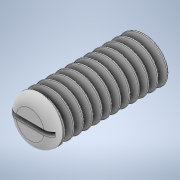
# Autodesk Inventor part: Tornillo de presion punta fuerte
Saved by Autodesk Inventor 2020 (Build 240168000, 168)
## iProperties
Created: 2020-09-17
Part Number: Tornillo de presion punta fuerte
Material: Generic
Document SubType Name: Modeling
Designer: aaron
Density: 1 g/cm^3
Appearance: Default
Author: aaron
Autodesk Inventor part; units mm, degrees
ref_plane "YZ Plane" through (0, 0, 0) normal (1, 0, 0) x (0, 1, 0)
ref_plane "XZ Plane" through (0, 0, 0) normal (0, 1, 0) x (-1, 0, 0)
ref_plane "XY Plane" through (0, 0, 0) normal (0, 0, 1) x (1, 0, 0)
sketch "Sketch1" plane through (0, 0, 0) normal (0, 0, 1) x (1, 0, 0)
  circle A0 centre (0, 0) radius 3.175
  dimension "d0" = 6.35
  constraints: 1 centre point, 1 coincident
  measures "d0" diameter of A0
extrude "Extrusion1" add sketch "Sketch1" against normal blind 15.875
fillet "Fillet1" radius 1.27 1 edges at (-3.175, 0, 0)
thread "Thread1" size "1/4-20 UNC" class "2A" standard "ANSI Unified Screw Threads" full length
sketch "Sketch3" plane through (0, 0, -15.875) normal (1, 0, 0) x (0, 1, 0)
  line L0 (3.175, 0) -> (3.175, 14.605)
  line L1 (3.175, 14.605) -> (2.2333, 14.605)
  line L2 (2.2333, 14.605) -> (2.2333, 0)
  line L3 (2.2333, 0) -> (3.175, 0)
  line L4 (0, -4.8369) -> (0, 19.327) projected
  constraints: 8 end point
revolve "Revolution1" cut sketch "Sketch3" angle 360 about axis through (0, 0, -15.875) along (0, 0, 1)
sketch "Sketch4" plane through (0, 0, -15.875) normal (1, 0, 0) x (0, 1, 0)
  line L0 (3.175, 0) -> (3.175, 14.605)
  line L1 (3.175, 14.605) -> (2.2333, 14.605)
  line L2 (2.2333, 14.605) -> (2.2333, 0)
  line L3 (2.2333, 0) -> (3.175, 0)
  line L4 (0, -4.8369) -> (0, 19.327) projected
  constraints: 8 end point
revolve "Revolution2" add sketch "Sketch4" angle 360 about axis through (0, 0, -15.875) along (0, 0, 1) separate body
sketch "Sketch2" plane through (0, 0, -15.875) normal (-1, 0, 0) x (0, 0, 1)
  line L0 (-0.7409, -2.2977) -> (-0.6351, -2.2977) construction
  line L1 (0.1057, -3.1109) -> (-0.0001, -3.3143) construction
  line L2 (-1.2701, -3.3143) -> (-1.3759, -3.1109) construction
  line L3 (-0.5293, -2.2977) -> (-0.6351, -2.0944) construction
  line L4 (-0.6351, -2.0944) -> (-0.7409, -2.2977) construction
  line L5 (-1.2701, -3.3143) -> (-1.1643, -3.1109) construction
  line L6 (-0.5293, -2.2977) -> (-0.1059, -3.1109)
  line L7 (-1.3759, -3.1109) -> (-1.1643, -3.1109) construction
  arc A0 (-1.3759, -3.1109) -> (-1.2701, -3.1752) centre (-1.2701, -3.0559) ccw construction
  line L8 (0.1057, -3.1109) -> (-0.1059, -3.1109) construction
  line L9 (-1.2701, -3.3143) -> (-1.2701, -3.1109) construction
  line L10 (-0.0001, -3.3143) -> (-0.0001, -3.1109) construction
  line L11 (-0.6351, -2.0944) -> (-0.6351, -2.2335) construction
  line L12 (-1.2701, -3.1752) -> (-0.0001, -3.1752)
  arc A1 (-1.2701, -3.1752) -> (-1.1643, -3.1109) centre (-1.2701, -3.0559) ccw
  line L13 (-0.1059, -3.1109) -> (-0.0001, -3.3143) construction
  line L14 (-1.1643, -3.1109) -> (-0.7409, -2.2977)
  line L15 (-0.0001, -0.0002) -> (-0.0001, 0.0177)
  line L16 (-0.0001, 0.0177) -> (-0.0001, -0.0002)
  line L17 (-0.0001, -0.0002) -> (0.0334, -0.0002)
  arc A2 (-0.1059, -3.1109) -> (-0.0001, -3.1752) centre (-0.0001, -3.0559) ccw
  arc A3 (-0.0001, -3.1752) -> (0.1057, -3.1109) centre (-0.0001, -3.0559) ccw construction
  arc A4 (-0.6351, -2.2335) -> (-0.7409, -2.2977) centre (-0.6351, -2.3528) ccw
  arc A5 (-0.5293, -2.2977) -> (-0.6351, -2.2335) centre (-0.6351, -2.3528) ccw
  line L18 (-0.6351, -2.2335) -> (-0.6351, -2.2977) construction
  line L19 (-0.6351, -2.2977) -> (-0.5293, -2.2977) construction
  dimension "d6" = 55
  dimension "d7" = 0.2033
  dimension "d8" = 0.2033
  dimension "Sketch2_ThreadOffset" = 0
  dimension "Sketch2_MajorRadius" = 3.175
  dimension "d11" = 1.27
  dimension "Sketch2_MinorRadius" = 2.2333
  constraints: 40 end point, 12 point on circle, 10 parallel, 8 tangent, 6 centre point, 6 collinear, 2 midpoint, 2 point on line, 1 horizontal, 1 perpendicular, 3 other
  measures "d6" angle of L6 L14
  measures "d7" distance of L3.end L0.end
  measures "d8" distance of L1.end L10.end
  measures "Sketch2_ThreadOffset" distance between parallel lines of L15 L10
  measures "Sketch2_MajorRadius" distance from line of L12 L15.start
  measures "d11" distance from line of L1.end L9
  measures "Sketch2_MinorRadius" distance edge to line of A5 L17
coil "Coil1" sketch "Sketch2" operation cut axis through (0, 0, -15.875) along (0, 0, 1) pitch 1.2713 turns 13.486513 hand right bodies 2
sketch "Sketch5" plane through (0, 0, 0) normal (0, 0, 1) x (1, 0, 0)
  line L0 (-2.9102, 0.3175) -> (2.9102, 0.3175)
  line L1 (2.9102, 0.3175) -> (2.9102, -0.3175)
  line L2 (2.9102, -0.3175) -> (-2.9102, -0.3175)
  line L3 (-2.9102, -0.3175) -> (-2.9102, 0.3175)
  line L4 (-2.9102, 0.3175) -> (2.9102, -0.3175) construction
  line L5 (2.9102, 0.3175) -> (-2.9102, -0.3175) construction
  point P0 (0, 0)
  dimension "d25" = 5.8204
  dimension "d26" = 0.635
  constraints: 12 end point, 2 midpoint, 2 parallel, 1 horizontal, 1 perpendicular
  measures "d25" distance of L0.start L0.end
  measures "d26" distance of L0.end L1.end
extrude "Extrusion2" cut sketch "Sketch5" against normal blind 1.27 bodies 1
equation "\"d6\" = d13"
equation "\"d7\" = 0.160083 * Sketch2_Pitch"
equation "\"d8\" = 0.160083 * Sketch2_Pitch"
equation "\"d11\" = Sketch2_Pitch"
equation "\"d13\" = 55deg"
equation "\"Sketch2_Pitch\" = 1.27"
body "Solid1"
body "Solid2"
